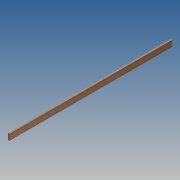
# Autodesk Inventor part: beam
Saved by Autodesk Inventor 2013 (Build 170138000, 138)
## iProperties
Created: 2013-08-10
Part Number: beam
Material: Wood (Birch)
Document SubType Name: Modeling
Designer: ddeboer
Mass: 14660.6 g
Surface Area: 15933.8 cm^2
Volume: 26655.6 cm^3
Density: 0.55 g/cm^3
Author: ddeboer
Autodesk Inventor part; units mm, degrees
ref_plane "YZ Plane" through (0, 0, 0) normal (1, 0, 0) x (0, 1, 0)
ref_plane "XZ Plane" through (0, 0, 0) normal (0, 1, 0) x (-1, 0, 0)
ref_plane "XY Plane" through (0, 0, 0) normal (0, 0, 1) x (1, 0, 0)
sketch "Sketch1" plane through (0, 0, 0) normal (0, 0, 1) x (1, 0, 0)
  line L0 (0, 0) -> (44.45, 0)
  line L1 (44.45, 0) -> (44.45, 190.5)
  line L2 (44.45, 190.5) -> (0, 190.5)
  line L3 (0, 190.5) -> (0, 0)
  dimension "d0" = 44.45
  dimension "d1" = 190.5
  constraints: 8 end point, 2 parallel, 1 horizontal, 1 perpendicular
  measures "d0" distance of L0.start L0.end
  measures "d1" distance of L2.end L0.start
extrude "Extrusion1" add sketch "Sketch1" along normal blind 5080
body "Solid1"
